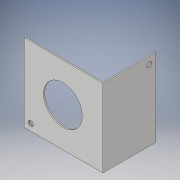
# Autodesk Inventor part: fixaçãoChaveGeral1
Saved by Autodesk Inventor 2019 (Build 230136000, 136)
## iProperties
Created: 2020-05-16
Part Number: fixaçãoChaveGeral1
Material: Genérico
Document SubType Name: Modeling
Designer: eliane
Density: 1 g/cm^3
Appearance: Padrão
Author: eliane
Autodesk Inventor part; units mm, degrees
ref_plane "YZ Plane" through (0, 0, 0) normal (1, 0, 0) x (0, 1, 0)
ref_plane "XZ Plane" through (0, 0, 0) normal (0, 1, 0) x (-1, 0, 0)
ref_plane "XY Plane" through (0, 0, 0) normal (0, 0, 1) x (1, 0, 0)
sketch "Esboço1" plane through (0, 0, 0) normal (0, 0, 1) x (1, 0, 0)
  circle A0 centre (0, 0) radius 22.5
  line L0 (0, 0) -> (-45, 0) construction
  line L1 (0, 0) -> (0, 45) construction
  line L2 (-45, 45) -> (45, 45)
  line L3 (45, 45) -> (45, -45)
  line L4 (45, -45) -> (-45, -45)
  line L5 (-45, -45) -> (-45, 45)
  dimension "d0" = 45
  dimension "d1" = 45
  dimension "d2" = 45
  dimension "d3" = 90
  dimension "d4" = 90
  constraints: 12 end point, 2 horizontal, 2 parallel, 1 centre point, 1 coincident, 1 perpendicular, 1 vertical
  measures "d0" diameter of A0
  measures "d1" distance of L0.start L0.end
  measures "d2" distance of L0.start L1.end
  measures "d3" distance of L3.end L4.end
  measures "d4" distance of L2.end L3.end
extrude "Extrusão1" add sketch "Esboço1" along normal blind 1.5
sketch "Esboço2" plane through (0, 0, 1.5) normal (0, 0, 1) x (1, 0, 0)
  line L0 (45, 45) -> (-45, 45) construction
  line L1 (-45, 45) -> (-45, 37) construction
  line L2 (-45, 45) -> (-45, -45) construction
  line L3 (-45, 37) -> (-37, 37) construction
  point P0 (0, 0)
  dimension "d7" = 8
  dimension "d8" = 8
  constraints: 4 end point, 1 perpendicular, 1 point on line
  measures "d7" distance of L0.end L1.end
  measures "d8" distance of L1.end L3.end
hole "Furo1" at (-37, 37, 1.5) direction (0, 0, -1) diameter 6 depth 13.5 tip angle 118
sketch "Esboço3" plane through (45, -45, 0) normal (1, 0, 0) x (0, 0, -1)
  point P0 (0, 45)
sketch "Esboço4" plane through (45, -45, 0) normal (1, 0, 0) x (0, 0, -1)
  line L0 (-1.5, 0) -> (-1.5, 90) projected
  line L1 (-1.5, 90) -> (60, 90)
  line L2 (60, 90) -> (60, 0)
  line L3 (60, 0) -> (-1.5, 0)
  line L4 (-1.5, 0) -> (-1.5, 90)
  line L5 (60, 90) -> (60, 82) construction
  line L6 (60, 82) -> (52, 82) construction
  circle A0 centre (52, 82) radius 3
  point P0 (0, 45)
  dimension "d16" = 61.5
  dimension "d17" = 8
  dimension "d18" = 8
  dimension "d19" = 6
  constraints: 12 end point, 2 parallel, 2 perpendicular, 1 centre point, 1 coincident, 1 horizontal, 1 point on line
  measures "d16" distance of L2.end L3.end
  measures "d17" distance of L1.end L5.end
  measures "d18" distance of L5.end L6.end
  measures "d19" diameter of A0
extrude "Extrusão2" add sketch "Esboço4" along normal blind 1.5
sketch "Esboço5" plane through (0, 0, 1.5) normal (0, 0, 1) x (1, 0, 0)
  circle A0 centre (-37, 37) radius 3 projected
  circle A1 centre (-37, 37) radius 3
  point P0 (0, 0)
  constraints: 1 centre point, 1 coincident
extrude "Extrusão3" add sketch "Esboço5" against normal blind 1.5
sketch "Esboço6" plane through (0, 0, 1.5) normal (0, 0, 1) x (1, 0, 0)
  line L0 (-45, -45) -> (-45, 45) construction
  line L1 (-45, -45) -> (-45, -37) construction
  line L2 (-45, -37) -> (-37, -37) construction
  point P0 (0, 0)
  dimension "d24" = 8
  dimension "d25" = 8
  constraints: 4 end point, 1 perpendicular, 1 point on line
  measures "d24" distance of L0.start L1.end
  measures "d25" distance of L1.end L2.end
hole "Furo2" at (-37, -37, 1.5) direction (0, 0, -1) diameter 6 depth 13.5 tip angle 118
